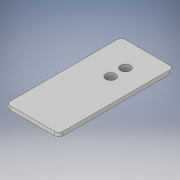
# Autodesk Inventor part: top
Saved by Autodesk Inventor 2017.3 (Build 213257000, 257)
## iProperties
Part Number: top
Material: Generisch
Document SubType Name: Modeling
Designer: Enno
Density: 1 g/cm^3
Appearance: Vorgabe
Author: Enno
Autodesk Inventor part; units mm, degrees
ref_plane "YZ Plane" through (0, 0, 0) normal (1, 0, 0) x (0, 1, 0)
ref_plane "XZ Plane" through (0, 0, 0) normal (0, 1, 0) x (-1, 0, 0)
ref_plane "XY Plane" through (0, 0, 0) normal (0, 0, 1) x (1, 0, 0)
sketch "Skizze1" plane through (0, 0, 0) normal (0, 0, 1) x (1, 0, 0)
  line L0 (0, 0) -> (27, 0)
  line L1 (27, 0) -> (27, 59)
  line L2 (27, 59) -> (0, 59)
  line L3 (0, 59) -> (0, 0)
  dimension "d0" = 27
  dimension "d1" = 59
  constraints: 8 end point, 2 parallel, 1 horizontal, 1 perpendicular
  measures "d0" distance of L1.end L2.end
  measures "d1" distance of L0.end L1.end
extrude "Extrusion1" add sketch "Skizze1" against normal blind 2
sketch "Skizze2" plane through (0, 0, -2) normal (0, 0, -1) x (-1, 0, 0)
  line L0 (-2, 2) -> (-25, 2)
  line L1 (-25, 2) -> (-25, 57)
  line L2 (-25, 57) -> (-2, 57)
  line L3 (-2, 57) -> (-2, 2)
  line L4 (0, 0) -> (0, 59) construction
  line L5 (-27, 0) -> (0, 0) construction
  point P0 (-2, 29.5)
  point P1 (0, 29.5)
  point P2 (-13.5, 2)
  point P3 (-13.5, 0)
  dimension "d4" = 2
  dimension "d5" = 2
  constraints: 8 end point, 4 midpoint, 2 parallel, 1 horizontal, 1 horizontal alignment, 1 perpendicular, 1 vertical alignment
  measures "d4" distance between parallel lines of L5 L0
  measures "d5" distance between parallel lines of L4 L3
extrude "Extrusion2" add sketch "Skizze2" along normal blind 2
sketch "Skizze3" plane through (0, 0, -4) normal (0, 0, -1) x (-1, 0, 0)
  circle A0 centre (-14.8, 38.8) radius 2.5
  line L0 (-27, 0) -> (0, 0) projected
  line L1 (-2, 2) -> (-2, 57) projected
  line L2 (-25, 57) -> (-25, 2) projected
  circle A1 centre (-14.8, 46.42) radius 2.5
  dimension "d8" = 5
  dimension "d9" = 38.8
  dimension "d11" = 10.2
  dimension "d12" = 5
  dimension "d13" = 7.62
  constraints: 2 centre point, 1 vertical alignment
  measures "d8" diameter of A0
  measures "d9" distance from line of L0 A0.centre
  measures "d11" distance from line of L2 A0.centre
  measures "d12" diameter of A1
  measures "d13" distance of A0.centre A1.centre
extrude "Extrusion3" cut sketch "Skizze3" against normal through all
fillet "Rundung1" radius 1 4 edges at (13.5, 57, -4) (25, 29.5, -4) (2, 29.5, -4) (13.5, 2, -4)
fillet "Rundung2" radius 2 4 edges at (0, 59, -1) (0, 0, -1) (27, 59, -1) (27, 0, -1)
